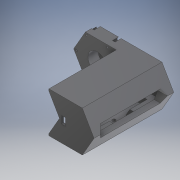
# Autodesk Inventor part: HA08
Saved by Autodesk Inventor 2017 (Build 210142000, 142)
## iProperties
Created: 2018-11-27
Part Number: HA08
Material: ABS Plastic
Document SubType Name: Modeling
Designer: Dell
Density: 1.06 g/cm^3
Appearance: Smooth - Black
Author: Dell
Autodesk Inventor part; units mm, degrees
ref_plane "YZ Plane" through (0, 0, 0) normal (1, 0, 0) x (0, 1, 0)
ref_plane "XZ Plane" through (0, 0, 0) normal (0, 1, 0) x (-1, 0, 0)
ref_plane "XY Plane" through (0, 0, 0) normal (0, 0, 1) x (1, 0, 0)
sketch "Sketch7" plane through (0, 0, 0) normal (0, 0, 1) x (1, 0, 0)
  line L0 (-57.5, 0) -> (-28.75, 49.7965)
  line L1 (-28.75, 49.7965) -> (28.75, 49.7965)
  line L2 (28.75, 49.7965) -> (57.5, 0)
  line L3 (57.5, 0) -> (28.75, -49.7965)
  line L4 (28.75, -49.7965) -> (-28.75, -49.7965)
  line L5 (-28.75, -49.7965) -> (-57.5, 0)
  circle A0 centre (0, 0) radius 22.5
  circle A1 centre (-51, 0) radius 2.5
  circle A2 centre (-25.5, -44.1673) radius 2.5
  circle A3 centre (25.5, -44.1673) radius 2.5
  circle A4 centre (51, 0) radius 2.5
  circle A5 centre (25.5, 44.1673) radius 2.5
  circle A6 centre (-25.5, 44.1673) radius 2.5
  line L6 (28.75, 49.7965) -> (157.5, 49.7965)
  line L7 (157.5, 49.7965) -> (157.5, -49.7965)
  line L8 (157.5, -49.7965) -> (28.75, -49.7965)
  dimension "d34" = 115
  dimension "d35" = 45
  dimension "d36" = 5
  dimension "d37" = 51
  dimension "d40" = 360
  dimension "d42" = 100
  constraints: 18 end point, 7 centre point, 2 coincident, 2 horizontal alignment, 2 perpendicular, 1 horizontal, 26 other
  measures "d34" distance of L2.end L0.start
  measures "d35" diameter of A0
  measures "d36" diameter of A1
  measures "d37" distance of A1.centre point (0, 0)
  measures "d42" distance from line of L7 L2.end
extrude "Extrusion7" add sketch "Sketch7" along normal blind 30
sketch "Sketch9" plane through (0, 0, 30) normal (0, 0, 1) x (1, 0, 0)
  line L0 (157.5, -49.7965) -> (157.5, 49.7965) projected
  line L1 (157.5, 0) -> (128.75, -49.7965)
  line L2 (128.75, -49.7965) -> (71.25, -49.7965)
  line L3 (71.25, -49.7965) -> (42.5, 0)
  line L4 (42.5, 0) -> (71.25, 49.7965)
  line L5 (71.25, 49.7965) -> (128.75, 49.7965)
  line L6 (128.75, 49.7965) -> (157.5, 0)
  line L7 (157.5, 49.7965) -> (-28.75, 49.7965) projected
  line L8 (-28.75, -49.7965) -> (157.5, -49.7965) projected
  line L9 (128.75, 49.7965) -> (157.5, 49.7965)
  line L10 (157.5, 49.7965) -> (157.5, 0)
  line L11 (157.5, 0) -> (157.5, -49.7965)
  line L12 (157.5, -49.7965) -> (128.75, -49.7965)
  point P0 (0, 0)
  point P1 (100, 0)
  point P2 (100, 49.7965)
  point P3 (100, -49.7965)
  constraints: 20 end point, 4 collinear, 3 midpoint, 2 point on line, 13 other
extrude "Extrusion8" cut sketch "Sketch9" against normal through all contours L8 L1 L0 | L6 L7 L0
sketch "Sketch10" plane through (0, 0, 30) normal (0, 0, 1) x (1, 0, 0)
  line L0 (157.5, 0) -> (128.75, 49.7965) projected
  line L1 (128.75, -49.7965) -> (157.5, 0) projected
  line L2 (-28.75, -49.7965) -> (128.75, -49.7965) projected
  line L3 (128.75, 49.7965) -> (-28.75, 49.7965) projected
  line L4 (128.75, 49.7965) -> (103.75, 49.7965)
  line L5 (128.75, 49.7965) -> (-28.75, 49.7965) projected
  line L6 (103.75, 49.7965) -> (132.5, 0)
  line L7 (132.5, 0) -> (103.75, -49.7965)
  line L8 (103.75, -49.7965) -> (128.75, -49.7965)
  point P0 (0, 0)
  dimension "d47" = 25
  constraints: 8 end point, 2 parallel, 2 point on line, 1 collinear, 1 horizontal alignment
  measures "d47" distance of L0.start L6.end
extrude "Extrusion9" add sketch "Sketch10" along normal blind 165
sketch "Sketch11" plane through (0, 0, 0) normal (1, 0, 0) x (0, 1, 0)
  line L0 (15, 179.5) -> (-15, 179.5)
  line L1 (-15, 179.5) -> (-15, 15.5)
  line L2 (-15, 15.5) -> (15, 15.5)
  line L3 (15, 15.5) -> (15, 179.5)
  line L4 (49.7965, 195) -> (49.7965, 0) projected
  line L5 (0, 179.5) -> (15, 170.8397)
  line L6 (15, 170.8397) -> (15, 153.5192)
  line L7 (15, 153.5192) -> (0, 144.859)
  line L8 (0, 144.859) -> (-15, 153.5192)
  line L9 (-15, 153.5192) -> (-15, 170.8397)
  line L10 (-15, 170.8397) -> (0, 179.5)
  line L11 (0, 15.5) -> (-15, 24.1603)
  line L12 (-15, 24.1603) -> (-15, 41.4808)
  line L13 (-15, 41.4808) -> (0, 50.141)
  line L14 (0, 50.141) -> (15, 41.4808)
  line L15 (15, 41.4808) -> (15, 24.1603)
  line L16 (15, 24.1603) -> (0, 15.5)
  line L17 (0, 179.5) -> (15, 179.5)
  line L18 (15, 179.5) -> (15, 170.8397)
  line L19 (0, 179.5) -> (-15, 179.5)
  line L20 (-15, 179.5) -> (-15, 170.8397)
  line L21 (-15, 24.1603) -> (-15, 15.5)
  line L22 (15, 15.5) -> (15, 24.1603)
  line L23 (0, 15.5) -> (15, 15.5)
  point P0 (0, 0)
  point P1 (15, 97.5)
  point P2 (49.7965, 97.5)
  point P3 (0, 195)
  point P4 (0, 162.1795)
  point P5 (0, 32.8205)
  dimension "d50" = 164
  dimension "d51" = 30
  constraints: 46 end point, 7 collinear, 4 midpoint, 4 point on line, 2 parallel, 1 horizontal, 1 horizontal alignment, 1 perpendicular, 1 vertical alignment, 26 other
  measures "d50" distance between parallel lines of L2 L0
  measures "d51" distance of L0.start L0.end
extrude "Extrusion10" cut sketch "Sketch11" along normal through all contours L5 L3 L7 L8 L1 L10 | L3 L14 L13 L1 L8 L7 | L3 L16 L11 L1 L13 L14
sketch "Sketch12" plane through (-28.75, -49.7965, 0) normal (0, -1, 0) x (1, 0, 0)
  line L0 (157.5, 72.5) -> (97.5, 72.5)
  line L1 (97.5, 72.5) -> (97.5, 122.5)
  line L2 (97.5, 122.5) -> (157.5, 122.5)
  line L3 (157.5, 122.5) -> (157.5, 72.5)
  line L4 (177.5897, 24.1603) -> (177.5897, 170.8397) projected
  line L5 (157.5, 0) -> (157.5, 195) projected
  point P0 (28.75, 0)
  point P1 (177.5897, 97.5)
  point P2 (157.5, 97.5)
  dimension "d54" = 60
  dimension "d55" = 50
  constraints: 8 end point, 3 midpoint, 2 parallel, 1 horizontal, 1 horizontal alignment, 1 perpendicular
  measures "d54" distance of L1.end L2.end
  measures "d55" distance of L0.end L1.end
extrude "Extrusion11" add sketch "Sketch12" against normal blind 15
sketch "Sketch13" plane through (-28.75, -34.7965, 0) normal (0, 1, 0) x (1, 0, 0)
  circle A0 centre (137.5, -97.5) radius 4
  line L0 (97.5, -72.5) -> (97.5, -122.5) projected
  line L1 (132.5, -30) -> (132.5, -195) projected
  point P0 (28.75, 0)
  point P1 (97.5, -97.5)
  dimension "d58" = 8
  dimension "d69" = 5
  constraints: 1 centre point, 1 horizontal alignment, 1 midpoint
  measures "d58" diameter of A0
  measures "d69" distance from line of L1 A0.centre
extrude "Extrusion12" cut sketch "Sketch13" against normal through all
sketch "Sketch14" plane through (-28.75, -34.7965, 0) normal (0, 1, 0) x (1, 0, 0)
  arc A0 (141.1603, -95.8868) -> (141.1603, -99.1132) centre (137.5, -97.5) ccw projected
  line L0 (141.1603, -72.5) -> (141.1603, -95.8868) projected
  line L1 (141.1603, -72.5) -> (97.5, -72.5) projected
  line L2 (97.5, -72.5) -> (97.5, -122.5) projected
  line L3 (97.5, -122.5) -> (141.1603, -122.5) projected
  line L4 (141.1603, -72.5) -> (162.5897, -72.5)
  line L5 (162.5897, -72.5) -> (162.5897, -122.5)
  line L6 (162.5897, -122.5) -> (141.1603, -122.5)
  line L7 (141.1603, -122.5) -> (141.1603, -72.5)
  line L8 (177.5897, -170.8397) -> (177.5897, -24.1603) projected
  line L9 (141.1603, -99.1132) -> (141.1603, -122.5) projected
  point P0 (28.75, 0)
  dimension "d62" = 15
  constraints: 8 end point, 2 parallel, 1 horizontal, 1 perpendicular
  measures "d62" distance between parallel lines of L8 L5
extrude "Extrusion13" cut sketch "Sketch14" along normal blind 30 contours L0 L4 L5 L6 L7
sketch "Sketch15" plane through (133.8397, -34.7965, 72.5) normal (-1, 0, 0) x (0, 0, 1)
  line L0 (-59, 52.2965) -> (109, 52.2965)
  line L1 (109, 52.2965) -> (109, 17.2965)
  line L2 (109, 17.2965) -> (-59, 17.2965)
  line L3 (-59, 17.2965) -> (-59, 52.2965)
  line L4 (98.3397, 49.7965) -> (-48.3397, 49.7965) projected
  point P0 (-72.5, 34.7965)
  point P1 (-57, 34.7965)
  point P2 (-59, 34.7965)
  point P3 (25, 49.7965)
  point P4 (25, 52.2965)
  dimension "d65" = 168
  dimension "d66" = 35
  constraints: 8 end point, 3 midpoint, 2 parallel, 1 horizontal, 1 horizontal alignment, 1 perpendicular, 1 vertical alignment
  measures "d65" distance of L0.start L0.end
  measures "d66" distance of L2.end L0.start
extrude "Extrusion14" cut sketch "Sketch15" along normal blind 125
sketch "Sketch17" plane through (-28.75, 49.7965, 30) normal (0, 1, 0) x (1, 0, 0)
  line L0 (132.5, -165) -> (157.5, -165) projected
  line L1 (0.75, 30) -> (5.75, 30) projected
  line L2 (157.5, -165) -> (0.75, -165)
  line L3 (0.75, -165) -> (0.75, 30)
  line L4 (0.75, 30) -> (157.5, 30)
  line L5 (157.5, 30) -> (157.5, -165)
  point P0 (28.75, 30)
  constraints: 8 end point, 2 parallel, 1 horizontal, 1 perpendicular
extrude "Extrusion15" add sketch "Sketch17" against normal blind 15
sketch "Sketch18" plane through (103.75, -49.7965, 72.5) normal (0, 0, -1) x (-1, 0, 0)
  line L0 (0, 0) -> (-8.6603, 15) projected
  line L1 (0, 0) -> (35, 0) projected
  line L2 (35, 0) -> (35, 15) projected
  line L3 (-8.6603, 15) -> (35, 15) projected
  point P0 (103.75, 49.7965)
extrude "Extrusion16" add sketch "Sketch18" along normal blind 50
sketch "Sketch20" plane through (-28.75, 49.7965, 30) normal (0, 1, 0) x (1, 0, 0)
  line L0 (5.75, 0) -> (0.75, 0) projected
  line L1 (141.1603, -165) -> (0.75, -165) projected
  line L2 (0.75, 0) -> (75.75, 0)
  line L3 (75.75, 0) -> (75.75, -165)
  line L4 (75.75, -165) -> (0.75, -165)
  line L5 (0.75, -165) -> (0.75, 0)
  line L6 (157.5, -165) -> (0.75, -165) projected
  point P0 (28.75, 30)
  dimension "d76" = 75
  constraints: 8 end point, 2 parallel, 2 point on line, 1 horizontal, 1 perpendicular
  measures "d76" distance between parallel lines of L5 L3
extrude "Extrusion18" cut sketch "Sketch20" against normal through all
chamfer "Chamfer1" distance 10 angle 45 1 edges at (47, 34.7965, 112.5)
sketch "Sketch22" plane through (-28.75, -49.7965, 0) normal (0, -1, 0) x (1, 0, 0)
  line L0 (75.75, 195) -> (75.75, 30) projected
  line L1 (157.5, 195) -> (75.75, 195) projected
  line L2 (0, 0) -> (157.5, 0) projected
  line L3 (75.75, 195) -> (157.5, 195)
  line L4 (157.5, 195) -> (157.5, 0)
  line L5 (157.5, 0) -> (75.75, 0)
  line L6 (75.75, 0) -> (75.75, 195)
  circle A0 centre (137.5, 97.5) radius 4 projected
  point P0 (28.75, 0)
  constraints: 8 end point, 2 parallel, 1 horizontal, 1 perpendicular
extrude "Extrusion19" add sketch "Sketch22" against normal blind 15
chamfer "Chamfer2" distance 10 angle 45 1 edges at (47, -34.7965, 112.5)
sketch "Sketch32" plane through (0, 0, 0) normal (0, 0, -1) x (-1, 0, 0)
  circle A0 centre (0, 0) radius 22.5 projected
  circle A1 centre (25.5, -44.1673) radius 2.5 projected
  circle A2 centre (25.5, -44.1673) radius 2.5
  circle A3 centre (51, 0) radius 2.5
  circle A4 centre (25.5, 44.1673) radius 2.5
  circle A5 centre (-25.5, 44.1673) radius 2.5
  circle A6 centre (-51, 0) radius 2.5
  circle A7 centre (-25.5, -44.1673) radius 2.5
  dimension "d107" = 360
  constraints: 6 centre point, 1 coincident, 1 concentric, 13 other
extrude "Extrusion27" add sketch "Sketch32" against normal blind 5 contours A0
extrude "Extrusion28" cut sketch "Sketch32" against normal through all contours A1 | A3 | A4 | A5 | A6 | A7
sketch "Sketch33" plane through (0, 0, 195) normal (0, 0, 1) x (1, 0, 0)
  line L0 (47, -44.7965) -> (57, -34.7965) projected
  line L1 (57, 34.7965) -> (47, 44.7965) projected
  line L2 (57, 34.7965) -> (63.8655, 27.931)
  line L3 (63.8655, 27.931) -> (91.7965, 0)
  line L4 (57, -34.7965) -> (47, -44.7965) projected
  line L5 (91.7965, 0) -> (57, -34.7965)
  line L6 (57, -34.7965) -> (112.4103, -34.7965) projected
  line L7 (122.3964, 17.5) -> (132.5, 0) projected
  line L8 (132.5, 0) -> (122.3964, -17.5) projected
  line L9 (112.4103, 34.7965) -> (57, 34.7965) projected
  line L10 (133.8397, -34.7965) -> (112.4103, -34.7965) projected
  line L11 (57, -34.7965) -> (112.4103, -34.7965)
  line L12 (122.3964, 17.5) -> (112.4103, 34.7965) projected
  line L13 (47, 44.7965) -> (57, 34.7965) projected
  line L14 (112.4103, 34.7965) -> (57, 34.7965)
  line L15 (132.5, 0) -> (112.4103, 34.7965)
  line L16 (132.5, 0) -> (112.4103, -34.7965)
  constraints: 14 end point, 5 collinear, 1 horizontal, 1 parallel
extrude "Extrusion29" add sketch "Sketch33" against normal blind 5
sketch "Sketch34" plane through (0, 0, 195) normal (0, 0, 1) x (1, 0, 0)
  line L0 (72.8632, 0) -> (47, -44.7965)
  line L1 (47, -44.7965) -> (-4.7265, -44.7965)
  line L2 (-4.7265, -44.7965) -> (-30.5897, 0)
  line L3 (-30.5897, 0) -> (-4.7265, 44.7965)
  line L4 (-4.7265, 44.7965) -> (47, 44.7965)
  line L5 (47, 44.7965) -> (72.8632, 0)
  line L6 (47, -49.7965) -> (47, -44.7965) projected
  line L7 (47, 49.7965) -> (47, 44.7965) projected
  line L8 (91.7965, 0) -> (47, 44.7965) projected
  line L9 (47, -44.7965) -> (91.7965, 0) projected
  point P0 (0, 0)
  point P1 (21.1368, 0)
  constraints: 12 end point, 13 other
extrude "Extrusion30" add sketch "Sketch34" against normal blind 5 contours L5 L8 L9 L0
sketch "Sketch35" plane through (0, 0, 0) normal (0, 0, -1) x (-1, 0, 0)
  circle A0 centre (0, 0) radius 22.5 construction
  circle A1 centre (51, 0) radius 2.5 construction
  circle A2 centre (51, 0) radius 6.5
  circle A3 centre (25.5, 44.1673) radius 6.5
  circle A4 centre (-25.5, 44.1673) radius 6.5
  circle A5 centre (-51, 0) radius 6.5
  circle A6 centre (-25.5, -44.1673) radius 6.5
  circle A7 centre (25.5, -44.1673) radius 6.5
  dimension "d117" = 13
  dimension "d120" = 360
  constraints: 6 centre point, 1 coincident, 13 other
  measures "d117" diameter of A2
extrude "Extrusion31" cut sketch "Sketch35" against normal blind 15
sketch "Sketch36" plane through (0, 0, 195) normal (0, 0, 1) x (1, 0, 0)
  line L0 (77.8632, 9) -> (87.8632, 9)
  line L1 (87.8632, 9) -> (87.8632, -9)
  line L2 (87.8632, -9) -> (77.8632, -9)
  line L3 (77.8632, -9) -> (77.8632, 9)
  point P0 (0, 0)
  point P1 (72.8632, 0)
  point P2 (77.8632, 0)
  dimension "d124" = 10
  dimension "d125" = 18
  dimension "d129" = 5
  constraints: 8 end point, 2 parallel, 1 horizontal, 1 horizontal alignment, 1 midpoint, 1 perpendicular
  measures "d124" distance of L1.end L2.end
  measures "d125" distance of L0.end L1.end
  measures "d129" distance from line of point (72.863, 0) L3
extrude "Extrusion32" cut sketch "Sketch36" against normal blind 10
body "Solid2"
